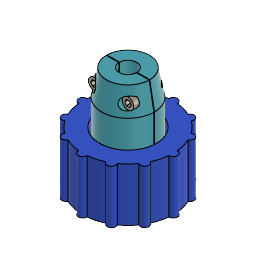
E80_connector (Autodesk Fusion 360 design; units mm, degrees)
Autodesk Fusion 360 part; units mm, degrees
ref_plane "WorkPlane7" through (0, 0, 0) normal (0, 0, 1) x (1, 0, 0)
ref_plane "WorkPlane8" through (0, 0, 5) normal (0, 0, 1) x (1, 0, 0)
ref_plane "WorkPlane9" through (0, 0, 12) normal (0, 0, 1) x (1, 0, 0)
ref_plane "WorkPlane11" through (0, 0, 14.8) normal (0, 0, 1) x (1, 0, 0)
ref_plane "WorkPlane12" through (0, 0, 28) normal (0, 0, 1) x (1, 0, 0)
ref_plane "WorkPlane13" through (0, 0, 37) normal (0, 0, 1) x (1, 0, 0)
sketch "main" plane through (0, 0, 0) normal (0, 0, 1) x (1, 0, 0)
  circle A0 centre (0, 0) radius 12.625
  line L0 (6, -4.5) -> (-6, 4.5) construction
  line L1 (-6, -4.5) -> (6, 4.5) construction
  circle A1 centre (0, 0) radius 3.1
  circle A2 centre (0, 0) radius 16
  line L2 (-1.25, 12.625) -> (-1.1331, 11.444)
  line L3 (1.25, 12.625) -> (1.1331, 11.444)
  line L4 (-1.25, -12.625) -> (-1.1331, -11.444)
  line L5 (1.25, -12.625) -> (1.1331, -11.444)
  arc A3 (-1.1331, -11.444) -> (1.1331, -11.444) centre (0, 0) ccw
  arc A4 (1.1331, 11.444) -> (-1.1331, 11.444) centre (0, 0) ccw
  arc A5 (1.4984, 15.9297) -> (-1.4984, 15.9297) centre (0, 16) ccw
  arc A6 (-6.6672, 14.5447) -> (-9.2625, 13.0463) centre (-8, 13.8564) ccw
  arc A7 (-13.0463, 9.2625) -> (-14.5447, 6.6672) centre (-13.8564, 8) ccw
  arc A8 (-15.9297, 1.4984) -> (-15.9297, -1.4984) centre (-16, 0) ccw
  arc A9 (-14.5447, -6.6672) -> (-13.0463, -9.2625) centre (-13.8564, -8) ccw
  arc A10 (-9.2625, -13.0463) -> (-6.6672, -14.5447) centre (-8, -13.8564) ccw
  arc A11 (-1.4984, -15.9297) -> (1.4984, -15.9297) centre (0, -16) ccw
  arc A12 (6.6672, -14.5447) -> (9.2625, -13.0463) centre (8, -13.8564) ccw
  arc A13 (13.0463, -9.2625) -> (14.5447, -6.6672) centre (13.8564, -8) ccw
  arc A14 (15.9297, -1.4984) -> (15.9297, 1.4984) centre (16, 0) ccw
  arc A15 (14.5447, 6.6672) -> (13.0463, 9.2625) centre (13.8564, 8) ccw
  arc A16 (9.2625, 13.0463) -> (6.6672, 14.5447) centre (8, 13.8564) ccw
  dimension "d1" = 25.25
  dimension "d2" = 23
  dimension "d4" = 12
  dimension "d5" = 9
  dimension "d6" = 6.2
  dimension "d7" = 32
  dimension "d11" = 360
  constraint coincident A0.centre A1.centre
  constraint concentric A0 A3
  constraint coincident L0 A0.centre
  constraint coincident L1 A0.centre
  constraint concentric A0 A1
  constraint coincident L3.end A3
  constraint concentric A3 A4
  constraint coincident A2 A5.centre
  constraint coincident A2 A5.end
  constraint coincident A2 A5.start
  measures "d1" diameter of A0
  measures "d2" diameter of A3
  measures "d4" distance of L0.end L1.end
  measures "d5" distance of L1.start L0.end
  measures "d6" diameter of A1
  measures "d7" diameter of A2
sketch "inner_bottom" plane through (0, 0, 5) normal (0, 0, 1) x (1, 0, 0)
  circle A0 centre (0, 0) radius 9.25
  circle A1 centre (0, 0) radius 3.1
  line L0 (6.1, 4.6) -> (-6.1, 4.6)
  line L1 (-6.1, 4.6) -> (-6.1, -4.6)
  line L2 (-6.1, -4.6) -> (6.1, -4.6)
  line L3 (6.1, -4.6) -> (6.1, 4.6)
  line L4 (6.1, 4.6) -> (-6.1, -4.6) construction
  line L5 (-6.1, 4.6) -> (6.1, -4.6) construction
  dimension "d62" = 18.5
  dimension "d83" = 6.2
  dimension "d84" = 12.2
  dimension "d85" = 9.2
  constraint horizontal L0
  constraint perpendicular L0 L1
  constraint parallel L0 L2
  constraint parallel L1 L3
  constraint coincident L4 A0.centre
  constraint coincident L5 A0.centre
  constraint coincident A0.centre A1.centre
  constraint midpoint A0.centre L4
  measures "d62" diameter of A0
  measures "d83" diameter of A1
  measures "d84" distance of L1.end L2.end
  measures "d85" distance of L0.end L1.end
sketch "upper" plane through (0, 0, 14.8) normal (0, 0, 1) x (1, 0, 0)
  circle A0 centre (0, 0) radius 16
  circle A1 centre (0, 0) radius 10
  constraint concentric A0 A1
sketch "cable_exit" plane through (0, 0, 37) normal (0, 0, 1) x (1, 0, 0)
  circle A0 centre (0, 0) radius 7.5788
  constraint coincident A0.centre origin
sketch "lower" plane through (0, 0, 12) normal (0, 0, 1) x (1, 0, 0)
  circle A0 centre (0, 0) radius 9.25
  circle A1 centre (0, 0) radius 12
  circle A2 centre (0, 0) radius 11.1
  line L0 (-1.8248, -10.949) -> (-1.9728, -11.8367)
  line L1 (1.9728, -11.8367) -> (1.8248, -10.949)
  line L2 (1.9728, 11.8367) -> (1.8248, 10.949)
  line L3 (-1.8248, 10.949) -> (-1.9728, 11.8367)
  constraint concentric A0 A1
  constraint concentric A1 A2
  constraint coincident A2 L0.start
  constraint coincident A1 L0.end
  constraint coincident A1 L1.start
  constraint coincident A2 L1.end
sketch "inner_top" plane through (0, 0, 28) normal (0, 0, 1) x (1, 0, 0)
  circle A0 centre (0, 0) radius 9.25
sketch "center" plane through (0, 0, 0) normal (0, 1, 0) x (-1, 0, 0)
  circle A0 centre (6, 32) radius 1.25
  circle A1 centre (6, 32) radius 0.9
  circle A2 centre (-6, 32) radius 0.9
  circle A3 centre (-6, 32) radius 1.25
  circle A4 centre (6, 32) radius 2
  circle A5 centre (-6, 32) radius 2
  line L0 (12, 12) -> (-12, 12) construction
  circle A6 centre (-10.3, 11) radius 1
  dimension "d67" = 2.5
  dimension "d68" = 1.8
  dimension "d69" = 2.5
  dimension "d70" = 1.8
  dimension "d94" = 4
  dimension "d95" = 4
  constraint concentric A0 A1
  constraint concentric A2 A3
  constraint concentric A0 A4
  constraint concentric A3 A5
  measures "d67" diameter of A0
  measures "d68" diameter of A1
  measures "d69" diameter of A3
  measures "d70" diameter of A2
  measures "d94" diameter of A4
  measures "d95" diameter of A5
extrude "Extrude11" add sketch "main" along normal blind 18.8 contours A2 | A2 A14 | A2 A15 | A2 A13 | A2 A16 | A2 A12 | A2 A5 | A2 A11 | A2 A6 | A2 A10 | A2 A7 | A2 A9 | A2 A8 makes body 1
extrude "Extrude12" add sketch "main" along normal blind 6.5 contours A0 L2 L3 A4 | A0 L4 L5 A3 bodies 1
extrude "Extrude13" add sketch "upper" along normal blind 4 bodies 1
loft "Loft1" add profiles "inner_top", "cable_exit" section 1 section 2 separate body makes body 2
extrude "Extrude14" add sketch "inner_bottom" along normal blind 23 contours A0 bodies 2
extrude "Extrude15" cut sketch "inner_bottom" along normal blind 41 contours A1 bodies 2
extrude "Extrude16" add sketch "lower" along normal blind 3 contours A1 A2 L1 L2 | A1 A2 L0 L3 | A2 bodies 2
split "Split2" by plane through (0, 0, 0) normal (0, 1, 0) bodies 2 makes body 3 at (-7.0859, 5.9458, 19.3333)
extrude "Extrude19" cut sketch "center" along normal blind 8 contours A1 | A2 bodies 3
extrude "Extrude20" cut sketch "center" against normal blind 8 contours A0 | A1 | A2 | A3 bodies 2
extrude "Extrude21" cut sketch "center" along normal blind -4 and the other way blind 16 contours A4 | A5 bodies 2
move_face "OffsetFaces4" offset -0.1 2 faces at (-7.15, 0, 16) (7.15, 0, 16) on bodies 3
move_face "OffsetFaces5" offset -0.1 2 faces at (-7.15, 0, 16) (7.15, 0, 16) on bodies 2
sketch "shaft_diam" plane through (0, 0, 0) normal (0, 0, 1) x (1, 0, 0) in component "hex_screw_M2x12 v1"
  circle A0 centre (0, 0) radius 1
  dimension "d4_1" = 2
  constraint coincident A0.centre origin
  measures "d4_1" diameter of A0
sketch "hex_head" plane through (0, 0, 0) normal (0, 0, 1) x (1, 0, 0) in component "hex_screw_M2x12 v1"
  circle A0 centre (0, 0) radius 2
  line L0 (-0.5774, 1) -> (-1.1547, 0)
  line L1 (-1.1547, 0) -> (-0.5774, -1)
  line L2 (-0.5774, -1) -> (0.5774, -1)
  line L3 (0.5774, -1) -> (1.1547, 0)
  line L4 (1.1547, 0) -> (0.5774, 1)
  line L5 (0.5774, 1) -> (-0.5774, 1)
  dimension "d7_1" = 4
  dimension "d8" = 1
  constraint coincident A0.centre origin
  measures "d7_1" diameter of A0
  measures "d8" distance of A0.centre L5
extrude "Extrude1" add sketch "shaft_diam" against normal blind 8 separate body makes body 4 in component "hex_screw_M2x12 v1"
extrude "Extrude2" add sketch "hex_head" along normal blind 2 separate body makes body 5 in component "hex_screw_M2x12 v1"
extrude "Extrude3" add sketch "hex_head" along normal blind 0.5 contours L0 L1 L2 L3 L4 L5 bodies 5 in component "hex_screw_M2x12 v1"
thread "Thread1" "ISO Metric profile 2.0 M2x0.4 6g" major diameter 1.9335 minor diameter 1.478 pitch 0.4 angle 60 resizes the face on face at (0.9988, -0.0498, -5.3333) on bodies 4 in component "hex_screw_M2x12 v1"
sketch "shaft_diam (2)" plane through (0, 0, 0) normal (0, 0, 1) x (1, 0, 0) in component "hex_screw_M2x12 v1 (1)"
  circle A0 centre (0, 0) radius 1
  dimension "d4_1_1" = 2
  constraint coincident A0.centre origin
  measures "d4_1_1" diameter of A0
sketch "hex_head (2)" plane through (0, 0, 0) normal (0, 0, 1) x (1, 0, 0) in component "hex_screw_M2x12 v1 (1)"
  circle A0 centre (0, 0) radius 2
  line L0 (-0.5774, 1) -> (-1.1547, 0)
  line L1 (-1.1547, 0) -> (-0.5774, -1)
  line L2 (-0.5774, -1) -> (0.5774, -1)
  line L3 (0.5774, -1) -> (1.1547, 0)
  line L4 (1.1547, 0) -> (0.5774, 1)
  line L5 (0.5774, 1) -> (-0.5774, 1)
  dimension "d7_1_1" = 4
  dimension "d8_1" = 1
  constraint coincident A0.centre origin
  measures "d7_1_1" diameter of A0
  measures "d8_1" distance of A0.centre L5
extrude "Extrude1'" add sketch "shaft_diam (2)" against normal blind 8 separate body makes body 6 in component "hex_screw_M2x12 v1 (1)"
extrude "Extrude2'" add sketch "hex_head (2)" along normal blind 2 separate body makes body 7 in component "hex_screw_M2x12 v1 (1)"
extrude "Extrude3'" add sketch "hex_head (2)" along normal blind 0.5 contours L0 L1 L2 L3 L4 L5 bodies 7 in component "hex_screw_M2x12 v1 (1)"
thread "Thread1'" "ISO Metric profile 2.0 M2x0.4 6g" major diameter 1.9335 minor diameter 1.478 pitch 0.4 angle 60 resizes the face on face at (0.9988, -0.0498, -5.3333) on bodies 6 in component "hex_screw_M2x12 v1 (1)"
revolve "Revolve1" add sketch "center" angle 360 about axis through (0, 0, 1.75) along (0, 0, 1) separate body contours A6 makes body 8 in component "oring"
component "hex_screw_M2x12 v1" placed x (1, 0, 0) y (0, 0, 1) z (0, -1, 0) at (6, -4, 32)
component "hex_screw_M2x12 v1 (1)" placed x (1, 0, 0) y (0, 0, 1) z (0, -1, 0) at (-6, -4, 32)
component "oring" placed x (1, 0, 0) y (0, 1, 0) z (0, 0, 1) at (0, 0, 0)
equation "inside_face = 5 mm"
equation "to_o_ring = 5.5 mm"
equation "o_ring = 1.5 mm"
equation "inner_lip_thick = 3 mm"
equation "outer_lip_thick = 4 mm"
equation "plug_depth = 23 mm"
equation "plug_width = 12.2 mm"
equation "plug_height = 9.2 mm"
equation "cable_diam = 6.2 mm"
equation "inner_height = 23 mm"
equation "nub_height = 6.5 mm"
equation "d57 = inside_face"
equation "d58 = to_o_ring + o_ring"
equation "d60 = inner_lip_thick + tightness_offset"
equation "d61 = inner_height"
equation "inner_taper_height = 9 mm"
equation "d66 = inner_taper_height"
equation "d71 = inside_face + to_o_ring + o_ring + inner_lip_thick + tightness_offset + outer_lip_thick"
equation "d73 = nub_height"
equation "d81 = inner_lip_thick"
equation "d83 = cable_diam"
equation "d84 = plug_width"
equation "d85 = plug_height"
equation "tightness_offset = -0.2 mm"
equation "shaft_diam = 2 mm"
equation "length = 12 mm"
equation "head_diam = 4 mm"
equation "d4_1 = shaft_diam"
equation "hex_radius = 1 mm"
equation "head_depth = 2 mm"
equation "d7_1 = head_diam"
equation "d8 = hex_radius"
equation "d21 = head_depth"
equation "d23 = head_depth / 4"
equation "d4_1_1 = shaft_diam"
equation "d7_1_1 = head_diam"
equation "d8_1 = hex_radius"
equation "d21_1 = head_depth"
equation "d23_1 = head_depth / 4"
named bodies: "shaft", "hex_head"
